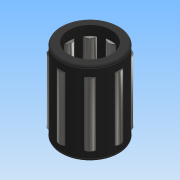
# Autodesk Inventor part: роликовый подшипник
Saved by Autodesk Inventor 2017 (Build 210142000, 142)
## iProperties
Part Number: роликовый подшипник
Material: Типовые
Document SubType Name: Modeling
Designer: STALKER
Density: 1 g/cm^3
Appearance: Сталь — полированная
Author: STALKER
Autodesk Inventor part; units mm, degrees
ref_plane "YZ Plane" through (0, 0, 0) normal (1, 0, 0) x (0, 1, 0)
ref_plane "XZ Plane" through (0, 0, 0) normal (0, 1, 0) x (-1, 0, 0)
ref_plane "XY Plane" through (0, 0, 0) normal (0, 0, 1) x (1, 0, 0)
sketch "Эскиз1" plane through (0, 0, 0) normal (0, 0, 1) x (1, 0, 0)
  circle A0 centre (0, 0) radius 2.4
  circle A1 centre (0, 0) radius 1.75
  circle A2 centre (0, 0) radius 1.5
  circle A3 centre (0, 0) radius 2.5
  line L0 (0, 0) -> (0, 4) construction
  circle A4 centre (0, 2) radius 0.5
  dimension "d0" = 4.8
  dimension "d1" = 3.5
  dimension "d2" = 3
  dimension "d3" = 5
  constraints: 5 centre point, 4 coincident, 2 end point, 1 midpoint
  measures "d0" diameter of A0
  measures "d1" diameter of A1
  measures "d2" diameter of A2
  measures "d3" diameter of A3
extrude "Выдавливание1" add sketch "Эскиз1" along normal mid plane 6.8 contours A0 A4 A1 | A4 A1 A0
extrude "Выдавливание2" add sketch "Эскиз1" along normal mid plane 5.2 contours A4 A1 A0 | A0 A4 | A1 A4 picked at (-0.2377, 2.1059) picked at (0, 1.6632)
pattern_circular "Круговой массив1" count 8 over 360 about axis through (0, 0, 0) along (0, 0, 1) of "Выдавливание2"
fillet "Сопряжение1" radius 0.2 2 edges at (-2.4, 0, 3.4) (-2.4, 0, -3.4)
